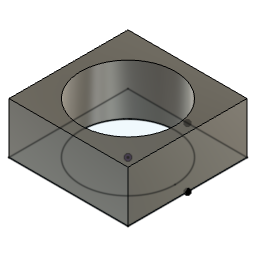
coupler (Autodesk Fusion 360 design; units mm, degrees)
Autodesk Fusion 360 part; units mm, degrees
sketch "Sketch1" plane through (0, 0, 0) normal (0, 0, 1) x (1, 0, 0)
  line L0 (-11.375, 11.375) -> (11.375, 11.375)
  line L1 (11.375, 11.375) -> (11.375, -11.375)
  line L2 (11.375, -11.375) -> (-11.375, -11.375)
  line L3 (-11.375, -11.375) -> (-11.375, 11.375)
  circle A0 centre (0, 0) radius 9
  point P0 (0, 11.375)
  point P1 (11.375, 0)
  dimension "d1" = 22.75
  dimension "d2" = 18
  constraint horizontal L0
  constraint vertical L1
  constraint horizontal L2
  constraint vertical L3
  constraint midpoint L0 P0
  constraint midpoint L1 P1
  constraint horizontal A0.centre P1
  constraint vertical A0.centre P0
  constraint equal L0 L3
  constraint coincident A0.centre origin
  measures "d1" distance of L0.start L0.end
  measures "d2" diameter of A0
extrude "Extrude3" add sketch "Sketch1" along normal blind 9.75
